WingedNutThroughScrewDouble2mm_v3 (Autodesk Fusion 360 design; units mm, degrees)
Autodesk Fusion 360 part; units mm, degrees
note: some values were not read from the file. Set by a fixed rule: which sketch regions a step uses.
sketch "Sketch1" plane through (0, 0, 0) normal (0, 0, 1) x (1, 0, 0)
  circle A0 centre (0, 0) radius 1.1
  circle A1 centre (0, 0) radius 2.15 construction
  line L0 (1.5877, -2.75) -> (3.1754, 0)
  line L1 (3.1754, 0) -> (1.5877, 2.75)
  line L2 (1.5877, 2.75) -> (-1.5877, 2.75)
  line L3 (-1.5877, 2.75) -> (-3.1754, 0)
  line L4 (-3.1754, 0) -> (-1.5877, -2.75)
  line L5 (-1.5877, -2.75) -> (1.5877, -2.75)
  circle A2 centre (-6, 0) radius 1.5
  circle A3 centre (-5.3127, -2.7883) radius 1.5
  circle A4 centre (-3.4084, -4.9379) radius 1.5
  circle A5 centre (-0.7232, -5.9563) radius 1.5
  circle A6 centre (2.1276, -5.6101) radius 1.5
  circle A7 centre (4.4911, -3.9787) radius 1.5
  circle A8 centre (5.8257, -1.4359) radius 1.5
  circle A9 centre (5.8257, 1.4359) radius 1.5
  circle A10 centre (4.4911, 3.9787) radius 1.5
  circle A11 centre (2.1276, 5.6101) radius 1.5
  circle A12 centre (-0.7232, 5.9563) radius 1.5
  circle A13 centre (-3.4084, 4.9379) radius 1.5
  circle A14 centre (-5.3127, 2.7883) radius 1.5
  line L6 (-1.2902, 2.2348) -> (-2.5805, 0)
  line L7 (-2.5805, 0) -> (-1.2902, -2.2348)
  line L8 (-1.2902, -2.2348) -> (1.2902, -2.2348)
  line L9 (1.2902, -2.2348) -> (2.5805, 0)
  line L10 (2.5805, 0) -> (1.2902, 2.2348)
  line L11 (1.2902, 2.2348) -> (-1.2902, 2.2348)
  circle A15 centre (-4.5, 0.0086) radius 0.75
  circle A16 centre (-0.0086, -4.5) radius 0.75
  circle A17 centre (4.5, -0.0086) radius 0.75
  circle A18 centre (0.0086, 4.5) radius 0.75
  circle A19 centre (29.8257, 1.4359) radius 1.5
  circle A20 centre (18.6873, 2.7883) radius 1.5
  circle A21 centre (20.5916, 4.9379) radius 1.5
  circle A22 centre (20.5916, -4.9379) radius 1.5
  circle A23 centre (28.4911, 3.9787) radius 1.5
  line L12 (22.7098, 2.2348) -> (21.4195, 0)
  circle A24 centre (26.1276, 5.6101) radius 1.5
  line L13 (25.5877, 2.75) -> (22.4123, 2.75)
  circle A25 centre (26.1276, -5.6101) radius 1.5
  circle A26 centre (18, 0) radius 1.5
  circle A27 centre (24, 0) radius 2.15 construction
  circle A28 centre (28.5, -0.0086) radius 0.75
  line L14 (22.7098, -2.2348) -> (25.2902, -2.2348)
  circle A29 centre (23.2768, -5.9563) radius 1.5
  line L15 (25.2902, 2.2348) -> (22.7098, 2.2348)
  circle A30 centre (19.5, 0.0086) radius 0.75
  circle A31 centre (29.8257, -1.4359) radius 1.5
  line L16 (27.1754, 0) -> (25.5877, 2.75)
  line L17 (22.4123, 2.75) -> (20.8246, 0)
  circle A32 centre (23.9914, -4.5) radius 0.75
  line L18 (25.5877, -2.75) -> (27.1754, 0)
  circle A33 centre (24.0086, 4.5) radius 0.75
  circle A34 centre (18.6873, -2.7883) radius 1.5
  line L19 (22.4123, -2.75) -> (25.5877, -2.75)
  circle A35 centre (24, 0) radius 1.1
  circle A36 centre (28.4911, -3.9787) radius 1.5
  circle A37 centre (23.2768, 5.9563) radius 1.5
  line L20 (21.4195, 0) -> (22.7098, -2.2348)
  line L21 (25.2902, -2.2348) -> (26.5805, 0)
  line L22 (20.8246, 0) -> (22.4123, -2.75)
  line L23 (26.5805, 0) -> (25.2902, 2.2348)
  point P0 (24, 0)
  point P1 (24, 0)
  dimension "d6" = 2.2
  dimension "d7" = 4.3
  dimension "d8" = 3
  dimension "d10" = 6
  dimension "d12" = 360
  dimension "d33" = 1.5
  dimension "d35" = 360
  dimension "d36" = 4.5
  dimension "d44" = 360
  dimension "d45" = 2.2
  dimension "d46" = 4.3
  dimension "d47" = 3
  dimension "d48" = 6
  dimension "d49" = 1.5
  dimension "d50" = 4.5
  constraint coincident A0.centre A1.centre
  constraint concentric A0 A1
  constraint concentric A27 A35
  measures "d6" diameter of A0
  measures "d7" diameter of A1
  measures "d8" diameter of A2
  measures "d10" distance of A0.centre A2.centre
  measures "d33" diameter of A15
  measures "d36" horizontal distance of A0.centre A15.centre
  measures "d45" diameter of A35
  measures "d46" diameter of A27
  measures "d47" diameter of A26
  measures "d48" distance of A26.centre P1
  measures "d49" diameter of A30
  measures "d50" horizontal distance of A30.centre P1
extrude "Extrude1" add sketch "Sketch1" along normal blind 3.1 contours A0 | L0 L1 L2 L3 L4 L5 | A2 A15 | A2 A15 | A2 A3 A14 A15 | A2 A3 A4 A5 A6 A7 A8 A9 A10 A11 A12 A13 A14 A15 A16 A17 A18 | A2 A14 | A2 A13 A14 | A2 A3 A4 | A2 A3 | A13 A14 | A12 A13 A14 | A3 A4 | A3 A4 A5 | A12 A13 | A11 A12 A13 A18 | A4 A5 | A4 A5 A6 A16 | A11 A12 | A10 A11 A12 | A5 A6 | A5 A6 A7 | A12 A18 | A12 A18 | A5 A16 | A5 A16 | A10 A11 | A9 A10 A11 | A6 A7 A8 | A6 A7 | A8 A9 A10 A17 | A9 A10 | A7 A8 A9 A17 | A7 A8 | A9 A17 | A8 A9 A17 | A8 A17 | A8 A9 A17 | A8 A9 | L6 L7 L8 L9 L10 L11 makes body 1
extrude "Extrude2" cut sketch "Sketch1" along normal blind 3.1 contours A0 bodies 1
extrude "Extrude3" cut sketch "Sketch1" along normal blind 1.6 from surface at 1.5 contours L0 L1 L2 L3 L4 L5 | L6 L7 L8 L9 L10 L11 bodies 1
copy_body "CopyPasteBodies2" bodies 1 makes body 2
move_body "Move2" bodies 2 to x (1, 0, 0) y (0, 1, 0) z (0, 0, 1) at (24, 0, 0)
extrude "Extrude5" add sketch "Sketch1" along normal blind 6.2 contours A2 A15 | A2 A15 | A12 A18 | A12 A18 | A5 A16 | A5 A16 | A9 A17 | A8 A9 A17 | A8 A17 picked at (4.4065, 0.0145) bodies 1
extrude "Extrude6" cut sketch "Sketch1" along normal blind 6.2 contours A19 A28 | A19 A28 A31 | A28 A31 | A33 A37 | A33 A37 | A29 A32 | A29 A32 | A26 A30 | A26 A30 picked at (28.4065, 0.0145) bodies 2
fillet "Fillet3" radius 0.4 4 edges at (-5.1992, -0.2626, 6.2) (-0.7079, -4.7712, 6.2) (-0.6906, 4.2288, 6.2) (3.8008, -0.2798, 6.2) on bodies 1
equation "screwDiam = 2.2 mm"
equation "FlatSideNutDistance = 4.3 mm"
equation "solidBaseHeight = 1.5 mm"
equation "nutHeight = 1.6 mm"
equation "wingDiameter = 12 mm"
equation "d6 = screwDiam"
equation "d7 = FlatSideNutDistance"
equation "d10 = wingDiameter / 2"
equation "d11 = bumpCicles"
equation "d12 = 360.00 °"
equation "bumpCicles = 13"
equation "d14 = nutHeight + solidBaseHeight"
equation "d16 = nutHeight + solidBaseHeight"
equation "d18 = solidBaseHeight"
equation "d19 = nutHeight"
equation "d35 = 360.0 °"
equation "d36 = wingDiameter / 2 - 1.5 mm"
equation "d41 = ( nutHeight + solidBaseHeight ) * 2"
equation "d44 = 360.0 °"
equation "d45 = screwDiam"
equation "d46 = FlatSideNutDistance"
equation "d48 = wingDiameter / 2"
equation "d50 = wingDiameter / 2 - 1.5 mm"
equation "d51 = ( nutHeight + solidBaseHeight ) * 2"
named bodies: "wing", "wing (1)"
